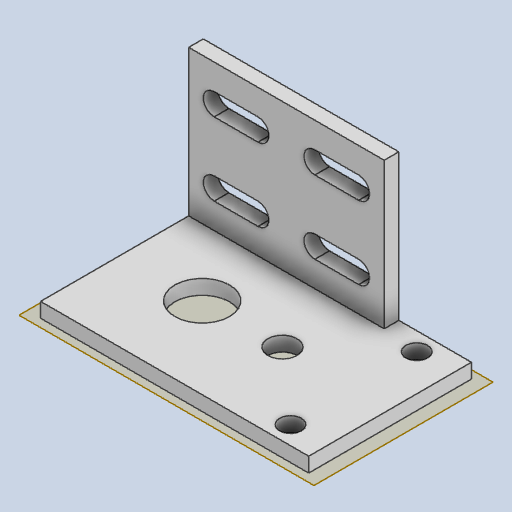
# Autodesk Inventor part: suporte_motor_amarelo
Saved by Autodesk Inventor 2023 (Build 270158000, 158)
## iProperties
Created: 2022-09-27
Part Number: suporte_motor_amarelo
Material: Generic
Document SubType Name: Modeling
Designer: kleber
Density: 1 g/cm^3
Appearance: Default
Author: kleber
Autodesk Inventor part; units mm, degrees
ref_plane "YZ Plane" through (0, 0, 0) normal (1, 0, 0) x (0, 1, 0)
ref_plane "XZ Plane" through (0, 0, 0) normal (0, 1, 0) x (-1, 0, 0)
ref_plane "XY Plane" through (0, 0, 0) normal (0, 0, 1) x (1, 0, 0)
ref_plane "Work Plane2" through (-101.9029, -40.2, 5.7831) normal (0, 1, 0) x (-1, 0, 0)
sketch "Sketch2" plane through (-101.9029, -40.2, 5.7831) normal (0, 1, 0) x (-1, 0, 0)
  circle A0 centre (8.0971, 5.3669) radius 3.75
  circle A1 centre (-2.9029, 5.3669) radius 2
  circle A2 centre (-12.6529, 14.0169) radius 1.5
  circle A3 centre (-12.6529, -3.2831) radius 1.5
  line L0 (-17.6529, 16.5169) -> (-17.6529, -5.7831)
  line L1 (-17.6529, -5.7831) -> (14.5971, -5.7831)
  line L2 (19.0971, -1.2831) -> (19.0971, 12.0169)
  line L3 (14.5971, 16.5169) -> (-17.6529, 16.5169)
  line L4 (-17.6529, 16.5169) -> (19.0971, 16.5169)
  line L5 (19.0971, 16.5169) -> (19.0971, -5.7831)
  line L6 (19.0971, -5.7831) -> (-17.6529, -5.7831)
  line L7 (-17.6529, -5.7831) -> (-17.6529, 16.5169)
  point P0 (-101.9029, -5.7831)
  point P1 (14.5971, -5.7831)
  point P2 (19.0971, -1.2831)
  point P3 (19.0971, 12.0169)
  constraints: 16 end point, 4 centre point, 2 parallel, 1 horizontal, 1 perpendicular
extrude "Extrusion2" add sketch "Sketch2" along normal blind 2
sketch "Sketch3" plane through (-101.9029, -38.2, 5.7831) normal (0, 1, 0) x (1, 0, 0)
  line L0 (17.6529, 5.7831) -> (-19.0971, 5.7831) projected
  line L1 (12.7, 3.175) -> (7.7, 3.175)
  line L2 (7.7, 3.175) -> (7.7, 5.7831)
  line L3 (7.7, 5.7831) -> (12.7, 5.7831)
  line L4 (12.7, 5.7831) -> (12.7, 3.175)
  line L5 (7.7, 5.7831) -> (-19.0971, 5.7831)
  line L6 (-19.0971, 5.7831) -> (-19.0971, 3.7831)
  line L7 (-19.0971, 3.7831) -> (7.7, 3.7831)
  line L8 (7.7, 3.7831) -> (7.7, 5.7831)
  point P0 (101.9029, 5.7831)
  point P1 (-14.5971, 5.7831)
  point P2 (7.7, 3.7831)
  dimension "d4" = 5
  dimension "d5" = 2
  constraints: 16 end point, 4 parallel, 2 horizontal, 2 perpendicular, 1 point on line
  measures "d4" distance of L2.end L3.end
  measures "d5" distance of L6.end L0.end
extrude "Extrusion3" add sketch "Sketch3" along normal blind 20 contours L2 L7 L6 L0
sketch "Sketch4" plane through (-121, -38.2, 2) normal (0, 0, 1) x (1, 0, 0)
  line L0 (26.7971, 0) -> (0, 0) projected
  line L1 (26.7971, 0) -> (26.7971, 20) projected
  line L2 (0, 20) -> (26.7971, 20) projected
  line L3 (0, 0) -> (0, 20) projected
  line L4 (18.7971, 16.5) -> (21.7971, 16.5)
  line L5 (18.7971, 16.5) -> (23.2971, 16.5)
  line L6 (23.2971, 13.5) -> (18.7971, 13.5)
  line L7 (18.7971, 3.5) -> (23.2971, 3.5)
  line L8 (23.2971, 6.5) -> (18.7971, 6.5)
  line L9 (3.5, 16.5) -> (5, 16.5)
  line L10 (3.5, 16.5) -> (8, 16.5)
  line L11 (8, 13.5) -> (3.5, 13.5)
  line L12 (3.5, 6.5) -> (5, 6.5)
  line L13 (3.5, 6.5) -> (8, 6.5)
  line L14 (8, 3.5) -> (3.5, 3.5)
  line L15 (18.7971, 3.5) -> (17.2971, 3.5)
  line L16 (17.2971, 6.5) -> (18.7971, 6.5)
  line L17 (8, 3.5) -> (9.5, 3.5)
  line L18 (9.5, 6.5) -> (8, 6.5)
  line L19 (18.7971, 13.5) -> (17.2971, 13.5)
  line L20 (17.2971, 16.5) -> (18.7971, 16.5)
  line L21 (8, 13.5) -> (9.5, 13.5)
  line L22 (9.5, 16.5) -> (8, 16.5)
  arc A0 (3.5, 6.5) -> (3.5, 3.5) centre (3.5, 5) ccw
  arc A1 (9.5, 3.5) -> (9.5, 6.5) centre (9.5, 5) ccw
  arc A2 (17.2971, 6.5) -> (17.2971, 3.5) centre (17.2971, 5) ccw
  arc A3 (23.2971, 3.5) -> (23.2971, 6.5) centre (23.2971, 5) ccw
  arc A4 (23.2971, 13.5) -> (23.2971, 16.5) centre (23.2971, 15) ccw
  arc A5 (17.2971, 16.5) -> (17.2971, 13.5) centre (17.2971, 15) ccw
  arc A6 (9.5, 13.5) -> (9.5, 16.5) centre (9.5, 15) ccw
  arc A7 (3.5, 16.5) -> (3.5, 13.5) centre (3.5, 15) ccw
  point P0 (121, 38.2)
  point P1 (18.7971, 6.5)
  point P2 (8, 6.5)
  point P3 (5, 6.5)
  point P4 (8, 16.5)
  point P5 (18.7971, 16.5)
  constraints: 38 end point, 16 point on circle, 16 tangent, 8 centre point, 7 horizontal, 7 parallel
extrude "Extrusion4" cut sketch "Sketch4" against normal through all contours L4 L5 A4 L6 L19 A5 L20 | L15 A2 L16 L8 A3 L7 | L9 L10 L22 A6 L21 L11 A7 | L12 L13 L18 A1 L17 L14 A0
body "Solid2"
